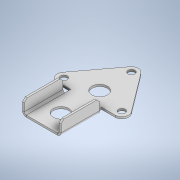
# Autodesk Inventor part: 26886-Vodička_Vojtěch_příklad-4
Saved by Autodesk Inventor 2022 (Build 260153000, 153)
## iProperties
Created: 2022-03-24
Part Number: 26886-Vodička_Vojtěch_příklad-4
Material: Všeobecné
Document SubType Name: Sheet Metal
Designer: vojta
Density: 1 g/cm^3
Sheet Metal Rule: Výchozí_mm
Appearance: Výchozí
Author: vojta
Autodesk Inventor part; units mm, degrees
ref_plane "YZ Plane" through (0, 0, 0) normal (1, 0, 0) x (0, 1, 0)
ref_plane "XZ Plane" through (0, 0, 0) normal (0, 1, 0) x (-1, 0, 0)
ref_plane "XY Plane" through (0, 0, 0) normal (0, 0, 1) x (1, 0, 0)
sketch "Náčrt1" plane through (0, 0, 0) normal (0, 1, 0) x (-1, 0, 0)
  line L0 (20, 0) -> (40, 0)
  line L1 (40, 0) -> (40, -40)
  line L2 (40, -40) -> (36, -40)
  line L3 (36, -40) -> (36, -46)
  circle A0 centre (50, -53) radius 3.5
  arc A1 (55.6, -57.2) -> (50, -46) centre (50, -53) ccw
  line L4 (36, -46) -> (50, -46)
  arc A2 (20, -96.5) -> (20, -89.5) centre (20, -93) ccw
  arc A3 (20, -100) -> (25.6, -97.2) centre (20, -93) ccw
  line L5 (55.6, -57.2) -> (25.6, -97.2)
  line L6 (20, 0) -> (0, 0)
  line L7 (0, 0) -> (0, -40)
  line L8 (0, -40) -> (4, -40)
  line L9 (4, -40) -> (4, -46)
  circle A4 centre (-10, -53) radius 3.5
  arc A5 (-10, -46) -> (-15.6, -57.2) centre (-10, -53) ccw
  line L10 (4, -46) -> (-10, -46)
  arc A6 (20, -89.5) -> (20, -96.5) centre (20, -93) ccw
  arc A7 (14.4, -97.2) -> (20, -100) centre (20, -93) ccw
  line L11 (-15.6, -57.2) -> (14.4, -97.2)
  dimension "d0" = 40
  dimension "d1" = 40
  dimension "d2" = 4
  dimension "d3" = 6
  dimension "d8" = 7
  dimension "d9" = 14
  dimension "d11" = 7
  dimension "d12" = 14
  dimension "d13" = 60
  measures "d0" distance of point (0, 0) L0.end
  measures "d1" distance of L0.end L1.end
  measures "d2" distance of L1.end L2.end
  measures "d3" distance of L2.end L3.end
  measures "d8" diameter of A0
  measures "d9" diameter of A1
  measures "d11" diameter of A2
  measures "d12" diameter of A3
  measures "d13" distance of A5.centre A0.centre
extrude "Deska1" add sketch "Náčrt1" along normal blind 2
sketch "Náčrt2" plane through (-38, 0, 0) normal (-1, 0, 0) x (0, -1, 0)
  line L0 (0, -40) -> (0, 0)
  line L1 (0, 0) -> (-15, 0)
  line L2 (-15, 0) -> (-15, -40)
  line L3 (-15, -40) -> (0, -40)
  constraints: 6 end point, 1 horizontal, 1 perpendicular, 1 vertical
edge flange "Obruba1" height 15 angle 90 thickness 2 bend radius 2 thickness toward (-1, 0, 0) relief tear relief width 2 relief depth 1 corner gap 2 corner form 0 edges at (-40, 2, -20) (0, 2, -20) wall of the first edge with corners at (-38, 0, -40) (-38, 0, 0) (-38, 15, 0) (-38, 15, -40)
bend "Ohyb1"
corner "Roh1"
chamfer "Zkosení rohu1" distance 3 angle 45 4 edges at (-39, 15, -40) (-39, 15, 0) (-1, 15, -40) (-1, 15, 0)
sketch "Náčrt3" plane through (0, 2, 0) normal (0, 1, 0) x (1, 0, 0)
  line L0 (-4, 0) -> (-36, 0) construction
  line L1 (-40, 40) -> (-40, 0) construction
  point P0 (0, 0)
  point P1 (-20, 20)
  dimension "d28" = 20
  dimension "d29" = 20
  measures "d28" distance from line of L0 point (-20, 20)
  measures "d29" distance from line of L1 point (-20, 20)
hole "Díra1" at (-20, 2, -20) direction (0, -1, 0) diameter 16 depth 2 tip angle 118
sketch "Náčrt5" plane through (0, 2, 0) normal (0, 1, 0) x (1, 0, 0)
  line L0 (-4, 0) -> (-36, 0) construction
  line L1 (-40, 37) -> (-40, 3) construction
  point P0 (0, 0)
  point P1 (-20, 60)
  dimension "d46" = 60
  dimension "d47" = 20
  measures "d46" distance from line of L0 point (-20, 60)
  measures "d47" distance from line of L1 point (-20, 60)
hole "Díra3" at (-20, 2, -60) direction (0, -1, 0) diameter 16 depth 2 tip angle 118
equation "\"d35\" = Tloušťka"
equation "\"d53\" = Tloušťka"
equation "\"d14\" = Tloušťka"
equation "\"d15\" = ŠířkaVýštipu"
equation "\"d16\" = HloubkaVýštipu"
equation "\"d17\" = MinimálníZbytek"
equation "\"d18\" = PřechodovýPoloměr"
equation "\"d21\" = PoloměrOhybu"
equation "\"d22\" = VelikostRohovéhoVýštipu"
equation "\"d23\" = VelikostMezery"
equation "\"d24\" = VelikostJacobihoPoloměru"
equation "\"PoloměrOhybu\" = Tloušťka"
equation "\"ŠířkaVýštipu\" = Tloušťka"
equation "\"HloubkaVýštipu\" = 0.5 * Tloušťka"
equation "\"VelikostRohovéhoVýštipu\" = 4 * Tloušťka"
equation "\"MinimálníZbytek\" = 2 * Tloušťka"
equation "\"PřechodovýPoloměr\" = PoloměrOhybu"
equation "\"VelikostJacobihoPoloměru\" = PoloměrOhybu"
equation "\"VelikostMezery\" = Tloušťka"
equation "\"Tloušťka\" = 2"
